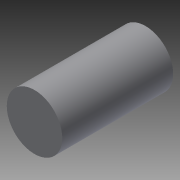
# Autodesk Inventor part: цевок10
Saved by Autodesk Inventor 2013 (Build 170138000, 138)
## iProperties
Created: 2014-04-30
Part Number: цевок10
Material: Типовые
Document SubType Name: Modeling
Designer: HP1
Density: 1 g/cm^3
Mass: 1.5708 g
Surface Area: 7.85398 cm^2
Volume: 1.5708 cm^3
Author: HP1
Autodesk Inventor part; units mm, degrees
ref_plane "YZ Plane" through (0, 0, 0) normal (1, 0, 0) x (0, 1, 0)
ref_plane "XZ Plane" through (0, 0, 0) normal (0, 1, 0) x (-1, 0, 0)
ref_plane "XY Plane" through (0, 0, 0) normal (0, 0, 1) x (1, 0, 0)
sketch "Эскиз1" plane through (0, 0, 0) normal (0, 1, 0) x (-1, 0, 0)
  circle A0 centre (0, 0) radius 5
  dimension "d0" = 10
  dimension "d0" = 10
  constraints: 1 centre point
  measures "d0" diameter of A0
extrude "Выдавливание1" add sketch "Эскиз1" along normal blind 20
